Autodesk Fusion 360 part; units mm, degrees
(part 2 of 12)
  line L834 (3.1315, 118.2846) -> (7.4616, 115.7846)
  line L835 (7.4616, 115.7846) -> (11.7918, 118.2846)
  line L836 (11.7918, 118.2846) -> (11.7918, 123.2846)
  line L837 (11.7918, 123.2846) -> (7.4616, 125.7846)
  line L838 (18.1219, 125.7846) -> (13.7918, 123.2846)
  line L839 (13.7918, 123.2846) -> (13.7918, 118.2846)
  line L840 (13.7918, 118.2846) -> (18.1219, 115.7846)
  line L841 (18.1219, 115.7846) -> (22.452, 118.2846)
  line L842 (22.452, 118.2846) -> (22.452, 123.2846)
  line L843 (22.452, 123.2846) -> (18.1219, 125.7846)
  line L844 (28.7821, 125.7846) -> (24.452, 123.2846)
  line L845 (24.452, 123.2846) -> (24.452, 118.2846)
  line L846 (24.452, 118.2846) -> (28.7821, 115.7846)
  line L847 (28.7821, 115.7846) -> (33.1123, 118.2846)
  line L848 (33.1123, 118.2846) -> (33.1123, 123.2846)
  line L849 (33.1123, 123.2846) -> (28.7821, 125.7846)
  line L850 (39.4424, 125.7846) -> (35.1123, 123.2846)
  line L851 (35.1123, 123.2846) -> (35.1123, 118.2846)
  line L852 (35.1123, 118.2846) -> (39.4424, 115.7846)
  line L853 (39.4424, 115.7846) -> (43.7725, 118.2846)
  line L854 (43.7725, 118.2846) -> (43.7725, 123.2846)
  line L855 (43.7725, 123.2846) -> (39.4424, 125.7846)
  line L856 (50.1027, 125.7846) -> (45.7725, 123.2846)
  line L857 (45.7725, 123.2846) -> (45.7725, 118.2846)
  line L858 (45.7725, 118.2846) -> (50.1027, 115.7846)
  line L859 (50.1027, 115.7846) -> (54.4328, 118.2846)
  line L860 (54.4328, 118.2846) -> (54.4328, 123.2846)
  line L861 (54.4328, 123.2846) -> (50.1027, 125.7846)
  line L862 (-51.1698, 135.0167) -> (-55.4999, 132.5167)
  line L863 (-55.4999, 132.5167) -> (-55.4999, 127.5167)
  line L864 (-55.4999, 127.5167) -> (-51.1698, 125.0167)
  line L865 (-51.1698, 125.0167) -> (-46.8396, 127.5167)
  line L866 (-46.8396, 127.5167) -> (-46.8396, 132.5167)
  line L867 (-46.8396, 132.5167) -> (-51.1698, 135.0167)
  line L868 (-40.5095, 135.0167) -> (-44.8396, 132.5167)
  line L869 (-44.8396, 132.5167) -> (-44.8396, 127.5167)
  line L870 (-44.8396, 127.5167) -> (-40.5095, 125.0167)
  line L871 (-40.5095, 125.0167) -> (-36.1794, 127.5167)
  line L872 (-36.1794, 127.5167) -> (-36.1794, 132.5167)
  line L873 (-36.1794, 132.5167) -> (-40.5095, 135.0167)
  line L874 (-29.8493, 135.0167) -> (-34.1794, 132.5167)
  line L875 (-34.1794, 132.5167) -> (-34.1794, 127.5167)
  line L876 (-34.1794, 127.5167) -> (-29.8493, 125.0167)
  line L877 (-29.8493, 125.0167) -> (-25.5191, 127.5167)
  line L878 (-25.5191, 127.5167) -> (-25.5191, 132.5167)
  line L879 (-25.5191, 132.5167) -> (-29.8493, 135.0167)
  line L880 (-19.189, 135.0167) -> (-23.5191, 132.5167)
  line L881 (-23.5191, 132.5167) -> (-23.5191, 127.5167)
  line L882 (-23.5191, 127.5167) -> (-19.189, 125.0167)
  line L883 (-19.189, 125.0167) -> (-14.8589, 127.5167)
  line L884 (-14.8589, 127.5167) -> (-14.8589, 132.5167)
  line L885 (-14.8589, 132.5167) -> (-19.189, 135.0167)
  line L886 (-8.5287, 135.0167) -> (-12.8589, 132.5167)
  line L887 (-12.8589, 132.5167) -> (-12.8589, 127.5167)
  line L888 (-12.8589, 127.5167) -> (-8.5287, 125.0167)
  line L889 (-8.5287, 125.0167) -> (-4.1986, 127.5167)
  line L890 (-4.1986, 127.5167) -> (-4.1986, 132.5167)
  line L891 (-4.1986, 132.5167) -> (-8.5287, 135.0167)
  line L892 (2.1315, 135.0167) -> (-2.1986, 132.5167)
  line L893 (-2.1986, 132.5167) -> (-2.1986, 127.5167)
  line L894 (-2.1986, 127.5167) -> (2.1315, 125.0167)
  line L895 (2.1315, 125.0167) -> (6.4616, 127.5167)
  line L896 (6.4616, 127.5167) -> (6.4616, 132.5167)
  line L897 (6.4616, 132.5167) -> (2.1315, 135.0167)
  line L898 (12.7918, 135.0167) -> (8.4616, 132.5167)
  line L899 (8.4616, 132.5167) -> (8.4616, 127.5167)
  line L900 (8.4616, 127.5167) -> (12.7918, 125.0167)
  line L901 (12.7918, 125.0167) -> (17.1219, 127.5167)
  line L902 (17.1219, 127.5167) -> (17.1219, 132.5167)
  line L903 (17.1219, 132.5167) -> (12.7918, 135.0167)
  line L904 (23.452, 135.0167) -> (19.1219, 132.5167)
  line L905 (19.1219, 132.5167) -> (19.1219, 127.5167)
  line L906 (19.1219, 127.5167) -> (23.452, 125.0167)
  line L907 (23.452, 125.0167) -> (27.7821, 127.5167)
  line L908 (27.7821, 127.5167) -> (27.7821, 132.5167)
  line L909 (27.7821, 132.5167) -> (23.452, 135.0167)
  line L910 (34.1123, 135.0167) -> (29.7821, 132.5167)
  line L911 (29.7821, 132.5167) -> (29.7821, 127.5167)
  line L912 (29.7821, 127.5167) -> (34.1123, 125.0167)
  line L913 (34.1123, 125.0167) -> (38.4424, 127.5167)
  line L914 (38.4424, 127.5167) -> (38.4424, 132.5167)
  line L915 (38.4424, 132.5167) -> (34.1123, 135.0167)
  line L916 (44.7725, 135.0167) -> (40.4424, 132.5167)
  line L917 (40.4424, 132.5167) -> (40.4424, 127.5167)
  line L918 (40.4424, 127.5167) -> (44.7725, 125.0167)
  line L919 (44.7725, 125.0167) -> (49.1027, 127.5167)
  line L920 (49.1027, 127.5167) -> (49.1027, 132.5167)
  line L921 (49.1027, 132.5167) -> (44.7725, 135.0167)
  line L922 (55.4328, 135.0167) -> (51.1027, 132.5167)
  line L923 (51.1027, 132.5167) -> (51.1027, 127.5167)
  line L924 (51.1027, 127.5167) -> (55.4328, 125.0167)
  line L925 (55.4328, 125.0167) -> (59.7629, 127.5167)
  line L926 (59.7629, 127.5167) -> (59.7629, 132.5167)
  line L927 (59.7629, 132.5167) -> (55.4328, 135.0167)
  line L928 (-56.4999, 144.2487) -> (-60.83, 141.7487)
  line L929 (-60.83, 141.7487) -> (-60.83, 136.7487)
  line L930 (-60.83, 136.7487) -> (-56.4999, 134.2487)
  line L931 (-56.4999, 134.2487) -> (-52.1698, 136.7487)
  line L932 (-52.1698, 136.7487) -> (-52.1698, 141.7487)
  line L933 (-52.1698, 141.7487) -> (-56.4999, 144.2487)
  line L934 (-45.8396, 144.2487) -> (-50.1698, 141.7487)
  line L935 (-50.1698, 141.7487) -> (-50.1698, 136.7487)
  line L936 (-50.1698, 136.7487) -> (-45.8396, 134.2487)
  line L937 (-45.8396, 134.2487) -> (-41.5095, 136.7487)
  line L938 (-41.5095, 136.7487) -> (-41.5095, 141.7487)
  line L939 (-41.5095, 141.7487) -> (-45.8396, 144.2487)
  line L940 (-35.1794, 144.2487) -> (-39.5095, 141.7487)
  line L941 (-39.5095, 141.7487) -> (-39.5095, 136.7487)
  line L942 (-39.5095, 136.7487) -> (-35.1794, 134.2487)
  line L943 (-35.1794, 134.2487) -> (-30.8493, 136.7487)
  line L944 (-30.8493, 136.7487) -> (-30.8493, 141.7487)
  line L945 (-30.8493, 141.7487) -> (-35.1794, 144.2487)
  line L946 (-24.5191, 144.2487) -> (-28.8493, 141.7487)
  line L947 (-28.8493, 141.7487) -> (-28.8493, 136.7487)
  line L948 (-28.8493, 136.7487) -> (-24.5191, 134.2487)
  line L949 (-24.5191, 134.2487) -> (-20.189, 136.7487)
  line L950 (-20.189, 136.7487) -> (-20.189, 141.7487)
  line L951 (-20.189, 141.7487) -> (-24.5191, 144.2487)
  line L952 (-13.8589, 144.2487) -> (-18.189, 141.7487)
  line L953 (-18.189, 141.7487) -> (-18.189, 136.7487)
  line L954 (-18.189, 136.7487) -> (-13.8589, 134.2487)
  line L955 (-13.8589, 134.2487) -> (-9.5287, 136.7487)
  line L956 (-9.5287, 136.7487) -> (-9.5287, 141.7487)
  line L957 (-9.5287, 141.7487) -> (-13.8589, 144.2487)
  line L958 (-3.1986, 144.2487) -> (-7.5287, 141.7487)
  line L959 (-7.5287, 141.7487) -> (-7.5287, 136.7487)
  line L960 (-7.5287, 136.7487) -> (-3.1986, 134.2487)
  line L961 (-3.1986, 134.2487) -> (1.1315, 136.7487)
  line L962 (1.1315, 136.7487) -> (1.1315, 141.7487)
  line L963 (1.1315, 141.7487) -> (-3.1986, 144.2487)
  line L964 (7.4616, 144.2487) -> (3.1315, 141.7487)
  line L965 (3.1315, 141.7487) -> (3.1315, 136.7487)
  line L966 (3.1315, 136.7487) -> (7.4616, 134.2487)
  line L967 (7.4616, 134.2487) -> (11.7918, 136.7487)
  line L968 (11.7918, 136.7487) -> (11.7918, 141.7487)
  line L969 (11.7918, 141.7487) -> (7.4616, 144.2487)
  line L970 (18.1219, 144.2487) -> (13.7918, 141.7487)
  line L971 (13.7918, 141.7487) -> (13.7918, 136.7487)
  line L972 (13.7918, 136.7487) -> (18.1219, 134.2487)
  line L973 (18.1219, 134.2487) -> (22.452, 136.7487)
  line L974 (22.452, 136.7487) -> (22.452, 141.7487)
  line L975 (22.452, 141.7487) -> (18.1219, 144.2487)
  line L976 (28.7821, 144.2487) -> (24.452, 141.7487)
  line L977 (24.452, 141.7487) -> (24.452, 136.7487)
  line L978 (24.452, 136.7487) -> (28.7821, 134.2487)
  line L979 (28.7821, 134.2487) -> (33.1123, 136.7487)
  line L980 (33.1123, 136.7487) -> (33.1123, 141.7487)
  line L981 (33.1123, 141.7487) -> (28.7821, 144.2487)
  line L982 (39.4424, 144.2487) -> (35.1123, 141.7487)
  line L983 (35.1123, 141.7487) -> (35.1123, 136.7487)
  line L984 (35.1123, 136.7487) -> (39.4424, 134.2487)
  line L985 (39.4424, 134.2487) -> (43.7725, 136.7487)
  line L986 (43.7725, 136.7487) -> (43.7725, 141.7487)
  line L987 (43.7725, 141.7487) -> (39.4424, 144.2487)
  line L988 (50.1027, 144.2487) -> (45.7725, 141.7487)
  line L989 (45.7725, 141.7487) -> (45.7725, 136.7487)
  line L990 (45.7725, 136.7487) -> (50.1027, 134.2487)
  line L991 (50.1027, 134.2487) -> (54.4328, 136.7487)
  line L992 (54.4328, 136.7487) -> (54.4328, 141.7487)
  line L993 (54.4328, 141.7487) -> (50.1027, 144.2487)
  line L994 (-51.1698, 153.4808) -> (-55.4999, 150.9808)
  line L995 (-55.4999, 150.9808) -> (-55.4999, 145.9808)
  line L996 (-55.4999, 145.9808) -> (-51.1698, 143.4808)
  line L997 (-51.1698, 143.4808) -> (-46.8396, 145.9808)
  line L998 (-46.8396, 145.9808) -> (-46.8396, 150.9808)
  line L999 (-46.8396, 150.9808) -> (-51.1698, 153.4808)
  line L1000 (-40.5095, 153.4808) -> (-44.8396, 150.9808)
  line L1001 (-44.8396, 150.9808) -> (-44.8396, 145.9808)
  line L1002 (-44.8396, 145.9808) -> (-40.5095, 143.4808)
  line L1003 (-40.5095, 143.4808) -> (-36.1794, 145.9808)
  line L1004 (-36.1794, 145.9808) -> (-36.1794, 150.9808)
  line L1005 (-36.1794, 150.9808) -> (-40.5095, 153.4808)
  line L1006 (-29.8493, 153.4808) -> (-34.1794, 150.9808)
  line L1007 (-34.1794, 150.9808) -> (-34.1794, 145.9808)
  line L1008 (-34.1794, 145.9808) -> (-29.8493, 143.4808)
  line L1009 (-29.8493, 143.4808) -> (-25.5191, 145.9808)
  line L1010 (-25.5191, 145.9808) -> (-25.5191, 150.9808)
  line L1011 (-25.5191, 150.9808) -> (-29.8493, 153.4808)
  line L1012 (-19.189, 153.4808) -> (-23.5191, 150.9808)
  line L1013 (-23.5191, 150.9808) -> (-23.5191, 145.9808)
  line L1014 (-23.5191, 145.9808) -> (-19.189, 143.4808)
  line L1015 (-19.189, 143.4808) -> (-14.8589, 145.9808)
  line L1016 (-14.8589, 145.9808) -> (-14.8589, 150.9808)
  line L1017 (-14.8589, 150.9808) -> (-19.189, 153.4808)
  line L1018 (-8.5287, 153.4808) -> (-12.8589, 150.9808)
  line L1019 (-12.8589, 150.9808) -> (-12.8589, 145.9808)
  line L1020 (-12.8589, 145.9808) -> (-8.5287, 143.4808)
  line L1021 (-8.5287, 143.4808) -> (-4.1986, 145.9808)
  line L1022 (-4.1986, 145.9808) -> (-4.1986, 150.9808)
  line L1023 (-4.1986, 150.9808) -> (-8.5287, 153.4808)
  line L1024 (2.1315, 153.4808) -> (-2.1986, 150.9808)
  line L1025 (-2.1986, 150.9808) -> (-2.1986, 145.9808)
  line L1026 (-2.1986, 145.9808) -> (2.1315, 143.4808)
  line L1027 (2.1315, 143.4808) -> (6.4616, 145.9808)
  line L1028 (6.4616, 145.9808) -> (6.4616, 150.9808)
  line L1029 (6.4616, 150.9808) -> (2.1315, 153.4808)
  line L1030 (12.7918, 153.4808) -> (8.4616, 150.9808)
  line L1031 (8.4616, 150.9808) -> (8.4616, 145.9808)
  line L1032 (8.4616, 145.9808) -> (12.7918, 143.4808)
  line L1033 (12.7918, 143.4808) -> (17.1219, 145.9808)
  line L1034 (17.1219, 145.9808) -> (17.1219, 150.9808)
  line L1035 (17.1219, 150.9808) -> (12.7918, 153.4808)
  line L1036 (23.452, 153.4808) -> (19.1219, 150.9808)
  line L1037 (19.1219, 150.9808) -> (19.1219, 145.9808)
  line L1038 (19.1219, 145.9808) -> (23.452, 143.4808)
  line L1039 (23.452, 143.4808) -> (27.7821, 145.9808)
  line L1040 (27.7821, 145.9808) -> (27.7821, 150.9808)
  line L1041 (27.7821, 150.9808) -> (23.452, 153.4808)
  line L1042 (34.1123, 153.4808) -> (29.7821, 150.9808)
  line L1043 (29.7821, 150.9808) -> (29.7821, 145.9808)
  line L1044 (29.7821, 145.9808) -> (34.1123, 143.4808)
  line L1045 (34.1123, 143.4808) -> (38.4424, 145.9808)
  line L1046 (38.4424, 145.9808) -> (38.4424, 150.9808)
  line L1047 (38.4424, 150.9808) -> (34.1123, 153.4808)
  line L1048 (44.7725, 153.4808) -> (40.4424, 150.9808)
  line L1049 (40.4424, 150.9808) -> (40.4424, 145.9808)
  line L1050 (40.4424, 145.9808) -> (44.7725, 143.4808)
  line L1051 (44.7725, 143.4808) -> (49.1027, 145.9808)
  line L1052 (49.1027, 145.9808) -> (49.1027, 150.9808)
  line L1053 (49.1027, 150.9808) -> (44.7725, 153.4808)
  line L1054 (55.4328, 153.4808) -> (51.1027, 150.9808)
  line L1055 (51.1027, 150.9808) -> (51.1027, 145.9808)
  line L1056 (51.1027, 145.9808) -> (55.4328, 143.4808)
  line L1057 (55.4328, 143.4808) -> (59.7629, 145.9808)
  line L1058 (59.7629, 145.9808) -> (59.7629, 150.9808)
  line L1059 (59.7629, 150.9808) -> (55.4328, 153.4808)
  line L1060 (-56.4999, 162.7128) -> (-60.83, 160.2128)
  line L1061 (-60.83, 160.2128) -> (-60.83, 155.2128)
  line L1062 (-60.83, 155.2128) -> (-56.4999, 152.7128)
  line L1063 (-56.4999, 152.7128) -> (-52.1698, 155.2128)
  line L1064 (-52.1698, 155.2128) -> (-52.1698, 160.2128)
  line L1065 (-52.1698, 160.2128) -> (-56.4999, 162.7128)
  line L1066 (-45.8396, 162.7128) -> (-50.1698, 160.2128)
  line L1067 (-50.1698, 160.2128) -> (-50.1698, 155.2128)
  line L1068 (-50.1698, 155.2128) -> (-45.8396, 152.7128)
  line L1069 (-45.8396, 152.7128) -> (-41.5095, 155.2128)
  line L1070 (-41.5095, 155.2128) -> (-41.5095, 160.2128)
  line L1071 (-41.5095, 160.2128) -> (-45.8396, 162.7128)
  line L1072 (-35.1794, 162.7128) -> (-39.5095, 160.2128)
  line L1073 (-39.5095, 160.2128) -> (-39.5095, 155.2128)
  line L1074 (-39.5095, 155.2128) -> (-35.1794, 152.7128)
  line L1075 (-35.1794, 152.7128) -> (-30.8493, 155.2128)
  line L1076 (-30.8493, 155.2128) -> (-30.8493, 160.2128)
  line L1077 (-30.8493, 160.2128) -> (-35.1794, 162.7128)
  line L1078 (-24.5191, 162.7128) -> (-28.8493, 160.2128)
  line L1079 (-28.8493, 160.2128) -> (-28.8493, 155.2128)
  line L1080 (-28.8493, 155.2128) -> (-24.5191, 152.7128)
  line L1081 (-24.5191, 152.7128) -> (-20.189, 155.2128)
  line L1082 (-20.189, 155.2128) -> (-20.189, 160.2128)
  line L1083 (-20.189, 160.2128) -> (-24.5191, 162.7128)
  line L1084 (-13.8589, 162.7128) -> (-18.189, 160.2128)
  line L1085 (-18.189, 160.2128) -> (-18.189, 155.2128)
  line L1086 (-18.189, 155.2128) -> (-13.8589, 152.7128)
  line L1087 (-13.8589, 152.7128) -> (-9.5287, 155.2128)
  line L1088 (-9.5287, 155.2128) -> (-9.5287, 160.2128)
  line L1089 (-9.5287, 160.2128) -> (-13.8589, 162.7128)
  line L1090 (-3.1986, 162.7128) -> (-7.5287, 160.2128)
  line L1091 (-7.5287, 160.2128) -> (-7.5287, 155.2128)
  line L1092 (-7.5287, 155.2128) -> (-3.1986, 152.7128)
  line L1093 (-3.1986, 152.7128) -> (1.1315, 155.2128)
  line L1094 (1.1315, 155.2128) -> (1.1315, 160.2128)
  line L1095 (1.1315, 160.2128) -> (-3.1986, 162.7128)
  line L1096 (7.4616, 162.7128) -> (3.1315, 160.2128)
  line L1097 (3.1315, 160.2128) -> (3.1315, 155.2128)
  line L1098 (3.1315, 155.2128) -> (7.4616, 152.7128)
  line L1099 (7.4616, 152.7128) -> (11.7918, 155.2128)
  line L1100 (11.7918, 155.2128) -> (11.7918, 160.2128)
  line L1101 (11.7918, 160.2128) -> (7.4616, 162.7128)
  line L1102 (18.1219, 162.7128) -> (13.7918, 160.2128)
  line L1103 (13.7918, 160.2128) -> (13.7918, 155.2128)
  line L1104 (13.7918, 155.2128) -> (18.1219, 152.7128)
  line L1105 (18.1219, 152.7128) -> (22.452, 155.2128)
  line L1106 (22.452, 155.2128) -> (22.452, 160.2128)
  line L1107 (22.452, 160.2128) -> (18.1219, 162.7128)
  line L1108 (28.7821, 162.7128) -> (24.452, 160.2128)
  line L1109 (24.452, 160.2128) -> (24.452, 155.2128)
  line L1110 (24.452, 155.2128) -> (28.7821, 152.7128)
  line L1111 (28.7821, 152.7128) -> (33.1123, 155.2128)
  line L1112 (33.1123, 155.2128) -> (33.1123, 160.2128)
  line L1113 (33.1123, 160.2128) -> (28.7821, 162.7128)
  line L1114 (39.4424, 162.7128) -> (35.1123, 160.2128)
  line L1115 (35.1123, 160.2128) -> (35.1123, 155.2128)
  line L1116 (35.1123, 155.2128) -> (39.4424, 152.7128)
  line L1117 (39.4424, 152.7128) -> (43.7725, 155.2128)
  line L1118 (43.7725, 155.2128) -> (43.7725, 160.2128)
  line L1119 (43.7725, 160.2128) -> (39.4424, 162.7128)
  line L1120 (50.1027, 162.7128) -> (45.7725, 160.2128)
  line L1121 (45.7725, 160.2128) -> (45.7725, 155.2128)
  line L1122 (45.7725, 155.2128) -> (50.1027, 152.7128)
  line L1123 (50.1027, 152.7128) -> (54.4328, 155.2128)
  line L1124 (54.4328, 155.2128) -> (54.4328, 160.2128)
  line L1125 (54.4328, 160.2128) -> (50.1027, 162.7128)
  line L1126 (-51.1698, 171.9449) -> (-55.4999, 169.4449)
  line L1127 (-55.4999, 169.4449) -> (-55.4999, 164.4449)
  line L1128 (-55.4999, 164.4449) -> (-51.1698, 161.9449)
  line L1129 (-51.1698, 161.9449) -> (-46.8396, 164.4449)
  line L1130 (-46.8396, 164.4449) -> (-46.8396, 169.4449)
  line L1131 (-46.8396, 169.4449) -> (-51.1698, 171.9449)
  line L1132 (-40.5095, 171.9449) -> (-44.8396, 169.4449)
  line L1133 (-44.8396, 169.4449) -> (-44.8396, 164.4449)
  line L1134 (-44.8396, 164.4449) -> (-40.5095, 161.9449)
  line L1135 (-40.5095, 161.9449) -> (-36.1794, 164.4449)
  line L1136 (-36.1794, 164.4449) -> (-36.1794, 169.4449)
  line L1137 (-36.1794, 169.4449) -> (-40.5095, 171.9449)
  line L1138 (-29.8493, 171.9449) -> (-34.1794, 169.4449)
  line L1139 (-34.1794, 169.4449) -> (-34.1794, 164.4449)
  line L1140 (-34.1794, 164.4449) -> (-29.8493, 161.9449)
  line L1141 (-29.8493, 161.9449) -> (-25.5191, 164.4449)
  line L1142 (-25.5191, 164.4449) -> (-25.5191, 169.4449)
  line L1143 (-25.5191, 169.4449) -> (-29.8493, 171.9449)
  line L1144 (-19.189, 171.9449) -> (-23.5191, 169.4449)
  line L1145 (-23.5191, 169.4449) -> (-23.5191, 164.4449)
  line L1146 (-23.5191, 164.4449) -> (-19.189, 161.9449)
  line L1147 (-19.189, 161.9449) -> (-14.8589, 164.4449)
  line L1148 (-14.8589, 164.4449) -> (-14.8589, 169.4449)
  line L1149 (-14.8589, 169.4449) -> (-19.189, 171.9449)
  line L1150 (-8.5287, 171.9449) -> (-12.8589, 169.4449)
  line L1151 (-12.8589, 169.4449) -> (-12.8589, 164.4449)
  line L1152 (-12.8589, 164.4449) -> (-8.5287, 161.9449)
  line L1153 (-8.5287, 161.9449) -> (-4.1986, 164.4449)
  line L1154 (-4.1986, 164.4449) -> (-4.1986, 169.4449)
  line L1155 (-4.1986, 169.4449) -> (-8.5287, 171.9449)
  line L1156 (2.1315, 171.9449) -> (-2.1986, 169.4449)
  line L1157 (-2.1986, 169.4449) -> (-2.1986, 164.4449)
  line L1158 (-2.1986, 164.4449) -> (2.1315, 161.9449)
  line L1159 (2.1315, 161.9449) -> (6.4616, 164.4449)
  line L1160 (6.4616, 164.4449) -> (6.4616, 169.4449)
  line L1161 (6.4616, 169.4449) -> (2.1315, 171.9449)
  line L1162 (12.7918, 171.9449) -> (8.4616, 169.4449)
  line L1163 (8.4616, 169.4449) -> (8.4616, 164.4449)
  line L1164 (8.4616, 164.4449) -> (12.7918, 161.9449)
  line L1165 (12.7918, 161.9449) -> (17.1219, 164.4449)
  line L1166 (17.1219, 164.4449) -> (17.1219, 169.4449)
  line L1167 (17.1219, 169.4449) -> (12.7918, 171.9449)
  line L1168 (23.452, 171.9449) -> (19.1219, 169.4449)
  line L1169 (19.1219, 169.4449) -> (19.1219, 164.4449)
  line L1170 (19.1219, 164.4449) -> (23.452, 161.9449)
  line L1171 (23.452, 161.9449) -> (27.7821, 164.4449)
  line L1172 (27.7821, 164.4449) -> (27.7821, 169.4449)
  line L1173 (27.7821, 169.4449) -> (23.452, 171.9449)
  line L1174 (34.1123, 171.9449) -> (29.7821, 169.4449)
  line L1175 (29.7821, 169.4449) -> (29.7821, 164.4449)
  line L1176 (29.7821, 164.4449) -> (34.1123, 161.9449)
  line L1177 (34.1123, 161.9449) -> (38.4424, 164.4449)
  line L1178 (38.4424, 164.4449) -> (38.4424, 169.4449)
  line L1179 (38.4424, 169.4449) -> (34.1123, 171.9449)
  line L1180 (44.7725, 171.9449) -> (40.4424, 169.4449)
  line L1181 (40.4424, 169.4449) -> (40.4424, 164.4449)
  line L1182 (40.4424, 164.4449) -> (44.7725, 161.9449)
  line L1183 (44.7725, 161.9449) -> (49.1027, 164.4449)
  line L1184 (49.1027, 164.4449) -> (49.1027, 169.4449)
  line L1185 (49.1027, 169.4449) -> (44.7725, 171.9449)
  line L1186 (55.4328, 171.9449) -> (51.1027, 169.4449)
  line L1187 (51.1027, 169.4449) -> (51.1027, 164.4449)
  line L1188 (51.1027, 164.4449) -> (55.4328, 161.9449)
  line L1189 (55.4328, 161.9449) -> (59.7629, 164.4449)
  line L1190 (59.7629, 164.4449) -> (59.7629, 169.4449)
  line L1191 (59.7629, 169.4449) -> (55.4328, 171.9449)
  line L1192 (-56.4999, 181.1769) -> (-60.83, 178.6769)
  line L1193 (-60.83, 178.6769) -> (-60.83, 173.6769)
  line L1194 (-60.83, 173.6769) -> (-56.4999, 171.1769)
  line L1195 (-56.4999, 171.1769) -> (-52.1698, 173.6769)
  line L1196 (-52.1698, 173.6769) -> (-52.1698, 178.6769)
  line L1197 (-52.1698, 178.6769) -> (-56.4999, 181.1769)
  line L1198 (-45.8396, 181.1769) -> (-50.1698, 178.6769)
  line L1199 (-50.1698, 178.6769) -> (-50.1698, 173.6769)
  line L1200 (-50.1698, 173.6769) -> (-45.8396, 171.1769)
  line L1201 (-45.8396, 171.1769) -> (-41.5095, 173.6769)
  line L1202 (-41.5095, 173.6769) -> (-41.5095, 178.6769)
  line L1203 (-41.5095, 178.6769) -> (-45.8396, 181.1769)
  line L1204 (-35.1794, 181.1769) -> (-39.5095, 178.6769)
  line L1205 (-39.5095, 178.6769) -> (-39.5095, 173.6769)
  line L1206 (-39.5095, 173.6769) -> (-35.1794, 171.1769)
  line L1207 (-35.1794, 171.1769) -> (-30.8493, 173.6769)
  line L1208 (-30.8493, 173.6769) -> (-30.8493, 178.6769)
  line L1209 (-30.8493, 178.6769) -> (-35.1794, 181.1769)
  line L1210 (-24.5191, 181.1769) -> (-28.8493, 178.6769)
  line L1211 (-28.8493, 178.6769) -> (-28.8493, 173.6769)
  line L1212 (-28.8493, 173.6769) -> (-24.5191, 171.1769)
  line L1213 (-24.5191, 171.1769) -> (-20.189, 173.6769)
  line L1214 (-20.189, 173.6769) -> (-20.189, 178.6769)
  line L1215 (-20.189, 178.6769) -> (-24.5191, 181.1769)
  line L1216 (-13.8589, 181.1769) -> (-18.189, 178.6769)
  line L1217 (-18.189, 178.6769) -> (-18.189, 173.6769)
  line L1218 (-18.189, 173.6769) -> (-13.8589, 171.1769)
  line L1219 (-13.8589, 171.1769) -> (-9.5287, 173.6769)
  line L1220 (-9.5287, 173.6769) -> (-9.5287, 178.6769)
  line L1221 (-9.5287, 178.6769) -> (-13.8589, 181.1769)
  line L1222 (-3.1986, 181.1769) -> (-7.5287, 178.6769)
  line L1223 (-7.5287, 178.6769) -> (-7.5287, 173.6769)
  line L1224 (-7.5287, 173.6769) -> (-3.1986, 171.1769)
  line L1225 (-3.1986, 171.1769) -> (1.1315, 173.6769)
  line L1226 (1.1315, 173.6769) -> (1.1315, 178.6769)
  line L1227 (1.1315, 178.6769) -> (-3.1986, 181.1769)
  line L1228 (7.4616, 181.1769) -> (3.1315, 178.6769)
  line L1229 (3.1315, 178.6769) -> (3.1315, 173.6769)
  line L1230 (3.1315, 173.6769) -> (7.4616, 171.1769)
  line L1231 (7.4616, 171.1769) -> (11.7918, 173.6769)
  line L1232 (11.7918, 173.6769) -> (11.7918, 178.6769)
  line L1233 (11.7918, 178.6769) -> (7.4616, 181.1769)
  line L1234 (18.1219, 181.1769) -> (13.7918, 178.6769)
  line L1235 (13.7918, 178.6769) -> (13.7918, 173.6769)
  line L1236 (13.7918, 173.6769) -> (18.1219, 171.1769)
  line L1237 (18.1219, 171.1769) -> (22.452, 173.6769)
  line L1238 (22.452, 173.6769) -> (22.452, 178.6769)
  line L1239 (22.452, 178.6769) -> (18.1219, 181.1769)
  line L1240 (28.7821, 181.1769) -> (24.452, 178.6769)
  line L1241 (24.452, 178.6769) -> (24.452, 173.6769)
  line L1242 (24.452, 173.6769) -> (28.7821, 171.1769)
  line L1243 (28.7821, 171.1769) -> (33.1123, 173.6769)
  line L1244 (33.1123, 173.6769) -> (33.1123, 178.6769)
  line L1245 (33.1123, 178.6769) -> (28.7821, 181.1769)
  line L1246 (39.4424, 181.1769) -> (35.1123, 178.6769)
  line L1247 (35.1123, 178.6769) -> (35.1123, 173.6769)
  line L1248 (35.1123, 173.6769) -> (39.4424, 171.1769)
  line L1249 (39.4424, 171.1769) -> (43.7725, 173.6769)
  line L1250 (43.7725, 173.6769) -> (43.7725, 178.6769)
  line L1251 (43.7725, 178.6769) -> (39.4424, 181.1769)
  line L1252 (50.1027, 181.1769) -> (45.7725, 178.6769)
  line L1253 (45.7725, 178.6769) -> (45.7725, 173.6769)
  line L1254 (45.7725, 173.6769) -> (50.1027, 171.1769)
  line L1255 (50.1027, 171.1769) -> (54.4328, 173.6769)
  line L1256 (54.4328, 173.6769) -> (54.4328, 178.6769)
  line L1257 (54.4328, 178.6769) -> (50.1027, 181.1769)
  line L1258 (-51.1698, 190.409) -> (-55.4999, 187.909)
  line L1259 (-55.4999, 187.909) -> (-55.4999, 182.909)
  line L1260 (-55.4999, 182.909) -> (-51.1698, 180.409)
  line L1261 (-51.1698, 180.409) -> (-46.8396, 182.909)
  line L1262 (-46.8396, 182.909) -> (-46.8396, 187.909)
  line L1263 (-46.8396, 187.909) -> (-51.1698, 190.409)
  line L1264 (-40.5095, 190.409) -> (-44.8396, 187.909)
  line L1265 (-44.8396, 187.909) -> (-44.8396, 182.909)
  line L1266 (-44.8396, 182.909) -> (-40.5095, 180.409)
  line L1267 (-40.5095, 180.409) -> (-36.1794, 182.909)
  line L1268 (-36.1794, 182.909) -> (-36.1794, 187.909)
  line L1269 (-36.1794, 187.909) -> (-40.5095, 190.409)
  line L1270 (-29.8493, 190.409) -> (-34.1794, 187.909)
  line L1271 (-34.1794, 187.909) -> (-34.1794, 182.909)
  line L1272 (-34.1794, 182.909) -> (-29.8493, 180.409)
  line L1273 (-29.8493, 180.409) -> (-25.5191, 182.909)
  line L1274 (-25.5191, 182.909) -> (-25.5191, 187.909)
  line L1275 (-25.5191, 187.909) -> (-29.8493, 190.409)
  line L1276 (-19.189, 190.409) -> (-23.5191, 187.909)
  line L1277 (-23.5191, 187.909) -> (-23.5191, 182.909)
  line L1278 (-23.5191, 182.909) -> (-19.189, 180.409)
  line L1279 (-19.189, 180.409) -> (-14.8589, 182.909)
  line L1280 (-14.8589, 182.909) -> (-14.8589, 187.909)
  line L1281 (-14.8589, 187.909) -> (-19.189, 190.409)
  line L1282 (-8.5287, 190.409) -> (-12.8589, 187.909)
  line L1283 (-12.8589, 187.909) -> (-12.8589, 182.909)
  line L1284 (-12.8589, 182.909) -> (-8.5287, 180.409)
  line L1285 (-8.5287, 180.409) -> (-4.1986, 182.909)
  line L1286 (-4.1986, 182.909) -> (-4.1986, 187.909)
  line L1287 (-4.1986, 187.909) -> (-8.5287, 190.409)
  line L1288 (2.1315, 190.409) -> (-2.1986, 187.909)
  line L1289 (-2.1986, 187.909) -> (-2.1986, 182.909)
  line L1290 (-2.1986, 182.909) -> (2.1315, 180.409)
  line L1291 (2.1315, 180.409) -> (6.4616, 182.909)
  line L1292 (6.4616, 182.909) -> (6.4616, 187.909)
  line L1293 (6.4616, 187.909) -> (2.1315, 190.409)
  line L1294 (12.7918, 190.409) -> (8.4616, 187.909)
  line L1295 (8.4616, 187.909) -> (8.4616, 182.909)
  line L1296 (8.4616, 182.909) -> (12.7918, 180.409)
  line L1297 (12.7918, 180.409) -> (17.1219, 182.909)
  line L1298 (17.1219, 182.909) -> (17.1219, 187.909)
  line L1299 (17.1219, 187.909) -> (12.7918, 190.409)
  line L1300 (23.452, 190.409) -> (19.1219, 187.909)
  line L1301 (19.1219, 187.909) -> (19.1219, 182.909)
  line L1302 (19.1219, 182.909) -> (23.452, 180.409)
  line L1303 (23.452, 180.409) -> (27.7821, 182.909)
  line L1304 (27.7821, 182.909) -> (27.7821, 187.909)
  line L1305 (27.7821, 187.909) -> (23.452, 190.409)
  line L1306 (34.1123, 190.409) -> (29.7821, 187.909)
  line L1307 (29.7821, 187.909) -> (29.7821, 182.909)
  line L1308 (29.7821, 182.909) -> (34.1123, 180.409)
  line L1309 (34.1123, 180.409) -> (38.4424, 182.909)
  line L1310 (38.4424, 182.909) -> (38.4424, 187.909)
  line L1311 (38.4424, 187.909) -> (34.1123, 190.409)
  line L1312 (44.7725, 190.409) -> (40.4424, 187.909)
  line L1313 (40.4424, 187.909) -> (40.4424, 182.909)
  line L1314 (40.4424, 182.909) -> (44.7725, 180.409)
  line L1315 (44.7725, 180.409) -> (49.1027, 182.909)
  line L1316 (49.1027, 182.909) -> (49.1027, 187.909)
  line L1317 (49.1027, 187.909) -> (44.7725, 190.409)
  line L1318 (55.4328, 190.409) -> (51.1027, 187.909)
  line L1319 (51.1027, 187.909) -> (51.1027, 182.909)
  line L1320 (51.1027, 182.909) -> (55.4328, 180.409)
  line L1321 (55.4328, 180.409) -> (59.7629, 182.909)
  line L1322 (59.7629, 182.909) -> (59.7629, 187.909)
  line L1323 (59.7629, 187.909) -> (55.4328, 190.409)
  line L1324 (-56.4999, 199.641) -> (-60.83, 197.141)
  line L1325 (-60.83, 197.141) -> (-60.83, 192.141)
  line L1326 (-60.83, 192.141) -> (-56.4999, 189.641)
  line L1327 (-56.4999, 189.641) -> (-52.1698, 192.141)
  line L1328 (-52.1698, 192.141) -> (-52.1698, 197.141)
  line L1329 (-52.1698, 197.141) -> (-56.4999, 199.641)
  line L1330 (-45.8396, 199.641) -> (-50.1698, 197.141)
  line L1331 (-50.1698, 197.141) -> (-50.1698, 192.141)
  line L1332 (-50.1698, 192.141) -> (-45.8396, 189.641)
  line L1333 (-45.8396, 189.641) -> (-41.5095, 192.141)
  line L1334 (-41.5095, 192.141) -> (-41.5095, 197.141)
  line L1335 (-41.5095, 197.141) -> (-45.8396, 199.641)
  line L1336 (-35.1794, 199.641) -> (-39.5095, 197.141)
  line L1337 (-39.5095, 197.141) -> (-39.5095, 192.141)
  line L1338 (-39.5095, 192.141) -> (-35.1794, 189.641)
  line L1339 (-35.1794, 189.641) -> (-30.8493, 192.141)
  line L1340 (-30.8493, 192.141) -> (-30.8493, 197.141)
  line L1341 (-30.8493, 197.141) -> (-35.1794, 199.641)
  line L1342 (-24.5191, 199.641) -> (-28.8493, 197.141)
  line L1343 (-28.8493, 197.141) -> (-28.8493, 192.141)
  line L1344 (-28.8493, 192.141) -> (-24.5191, 189.641)
  line L1345 (-24.5191, 189.641) -> (-20.189, 192.141)
  line L1346 (-20.189, 192.141) -> (-20.189, 197.141)
  line L1347 (-20.189, 197.141) -> (-24.5191, 199.641)
  line L1348 (-13.8589, 199.641) -> (-18.189, 197.141)
  line L1349 (-18.189, 197.141) -> (-18.189, 192.141)
  line L1350 (-18.189, 192.141) -> (-13.8589, 189.641)
  line L1351 (-13.8589, 189.641) -> (-9.5287, 192.141)
  line L1352 (-9.5287, 192.141) -> (-9.5287, 197.141)
  line L1353 (-9.5287, 197.141) -> (-13.8589, 199.641)
  line L1354 (-3.1986, 199.641) -> (-7.5287, 197.141)
  line L1355 (-7.5287, 197.141) -> (-7.5287, 192.141)
  line L1356 (-7.5287, 192.141) -> (-3.1986, 189.641)
  line L1357 (-3.1986, 189.641) -> (1.1315, 192.141)
  line L1358 (1.1315, 192.141) -> (1.1315, 197.141)
  line L1359 (1.1315, 197.141) -> (-3.1986, 199.641)
  line L1360 (7.4616, 199.641) -> (3.1315, 197.141)
  line L1361 (3.1315, 197.141) -> (3.1315, 192.141)
  line L1362 (3.1315, 192.141) -> (7.4616, 189.641)
  line L1363 (7.4616, 189.641) -> (11.7918, 192.141)
  line L1364 (11.7918, 192.141) -> (11.7918, 197.141)
  line L1365 (11.7918, 197.141) -> (7.4616, 199.641)
  line L1366 (18.1219, 199.641) -> (13.7918, 197.141)
  line L1367 (13.7918, 197.141) -> (13.7918, 192.141)
  line L1368 (13.7918, 192.141) -> (18.1219, 189.641)
  line L1369 (18.1219, 189.641) -> (22.452, 192.141)
  line L1370 (22.452, 192.141) -> (22.452, 197.141)
  line L1371 (22.452, 197.141) -> (18.1219, 199.641)
  line L1372 (28.7821, 199.641) -> (24.452, 197.141)
  line L1373 (24.452, 197.141) -> (24.452, 192.141)
  line L1374 (24.452, 192.141) -> (28.7821, 189.641)
  line L1375 (28.7821, 189.641) -> (33.1123, 192.141)
  line L1376 (33.1123, 192.141) -> (33.1123, 197.141)
  line L1377 (33.1123, 197.141) -> (28.7821, 199.641)
  line L1378 (39.4424, 199.641) -> (35.1123, 197.141)
  line L1379 (35.1123, 197.141) -> (35.1123, 192.141)
  line L1380 (35.1123, 192.141) -> (39.4424, 189.641)
  line L1381 (39.4424, 189.641) -> (43.7725, 192.141)
  line L1382 (43.7725, 192.141) -> (43.7725, 197.141)
  line L1383 (43.7725, 197.141) -> (39.4424, 199.641)
  line L1384 (50.1027, 199.641) -> (45.7725, 197.141)
  line L1385 (45.7725, 197.141) -> (45.7725, 192.141)
  line L1386 (45.7725, 192.141) -> (50.1027, 189.641)
  line L1387 (50.1027, 189.641) -> (54.4328, 192.141)
  line L1388 (54.4328, 192.141) -> (54.4328, 197.141)
  line L1389 (54.4328, 197.141) -> (50.1027, 199.641)
  line L1390 (-51.1698, 208.8731) -> (-55.4999, 206.3731)
  line L1391 (-55.4999, 206.3731) -> (-55.4999, 201.3731)
  line L1392 (-55.4999, 201.3731) -> (-51.1698, 198.8731)
  line L1393 (-51.1698, 198.8731) -> (-46.8396, 201.3731)
  line L1394 (-46.8396, 201.3731) -> (-46.8396, 206.3731)
  line L1395 (-46.8396, 206.3731) -> (-51.1698, 208.8731)
  line L1396 (-40.5095, 208.8731) -> (-44.8396, 206.3731)
  line L1397 (-44.8396, 206.3731) -> (-44.8396, 201.3731)
  line L1398 (-44.8396, 201.3731) -> (-40.5095, 198.8731)
  line L1399 (-40.5095, 198.8731) -> (-36.1794, 201.3731)
  line L1400 (-36.1794, 201.3731) -> (-36.1794, 206.3731)
  line L1401 (-36.1794, 206.3731) -> (-40.5095, 208.8731)
  line L1402 (-29.8493, 208.8731) -> (-34.1794, 206.3731)
  line L1403 (-34.1794, 206.3731) -> (-34.1794, 201.3731)
  line L1404 (-34.1794, 201.3731) -> (-29.8493, 198.8731)
  line L1405 (-29.8493, 198.8731) -> (-25.5191, 201.3731)
  line L1406 (-25.5191, 201.3731) -> (-25.5191, 206.3731)
  line L1407 (-25.5191, 206.3731) -> (-29.8493, 208.8731)
  line L1408 (-19.189, 208.8731) -> (-23.5191, 206.3731)
  line L1409 (-23.5191, 206.3731) -> (-23.5191, 201.3731)
  line L1410 (-23.5191, 201.3731) -> (-19.189, 198.8731)
  line L1411 (-19.189, 198.8731) -> (-14.8589, 201.3731)
  line L1412 (-14.8589, 201.3731) -> (-14.8589, 206.3731)
  line L1413 (-14.8589, 206.3731) -> (-19.189, 208.8731)
  line L1414 (-8.5287, 208.8731) -> (-12.8589, 206.3731)
  line L1415 (-12.8589, 206.3731) -> (-12.8589, 201.3731)
  line L1416 (-12.8589, 201.3731) -> (-8.5287, 198.8731)
  line L1417 (-8.5287, 198.8731) -> (-4.1986, 201.3731)
  line L1418 (-4.1986, 201.3731) -> (-4.1986, 206.3731)
  line L1419 (-4.1986, 206.3731) -> (-8.5287, 208.8731)
  line L1420 (2.1315, 208.8731) -> (-2.1986, 206.3731)
  line L1421 (-2.1986, 206.3731) -> (-2.1986, 201.3731)
  line L1422 (-2.1986, 201.3731) -> (2.1315, 198.8731)
  line L1423 (2.1315, 198.8731) -> (6.4616, 201.3731)
  line L1424 (6.4616, 201.3731) -> (6.4616, 206.3731)
  line L1425 (6.4616, 206.3731) -> (2.1315, 208.8731)
  line L1426 (12.7918, 208.8731) -> (8.4616, 206.3731)
  line L1427 (8.4616, 206.3731) -> (8.4616, 201.3731)
  line L1428 (8.4616, 201.3731) -> (12.7918, 198.8731)
  line L1429 (12.7918, 198.8731) -> (17.1219, 201.3731)
  line L1430 (17.1219, 201.3731) -> (17.1219, 206.3731)
  line L1431 (17.1219, 206.3731) -> (12.7918, 208.8731)
  line L1432 (23.452, 208.8731) -> (19.1219, 206.3731)
  line L1433 (19.1219, 206.3731) -> (19.1219, 201.3731)
  line L1434 (19.1219, 201.3731) -> (23.452, 198.8731)
  line L1435 (23.452, 198.8731) -> (27.7821, 201.3731)
  line L1436 (27.7821, 201.3731) -> (27.7821, 206.3731)
  line L1437 (27.7821, 206.3731) -> (23.452, 208.8731)
  line L1438 (34.1123, 208.8731) -> (29.7821, 206.3731)
  line L1439 (29.7821, 206.3731) -> (29.7821, 201.3731)
  line L1440 (29.7821, 201.3731) -> (34.1123, 198.8731)
  line L1441 (34.1123, 198.8731) -> (38.4424, 201.3731)
  line L1442 (38.4424, 201.3731) -> (38.4424, 206.3731)
  line L1443 (38.4424, 206.3731) -> (34.1123, 208.8731)
  line L1444 (44.7725, 208.8731) -> (40.4424, 206.3731)
  line L1445 (40.4424, 206.3731) -> (40.4424, 201.3731)
  line L1446 (40.4424, 201.3731) -> (44.7725, 198.8731)
  line L1447 (44.7725, 198.8731) -> (49.1027, 201.3731)
  line L1448 (49.1027, 201.3731) -> (49.1027, 206.3731)
  line L1449 (49.1027, 206.3731) -> (44.7725, 208.8731)
  line L1450 (55.4328, 208.8731) -> (51.1027, 206.3731)
  line L1451 (51.1027, 206.3731) -> (51.1027, 201.3731)
  line L1452 (51.1027, 201.3731) -> (55.4328, 198.8731)
  line L1453 (55.4328, 198.8731) -> (59.7629, 201.3731)
  line L1454 (59.7629, 201.3731) -> (59.7629, 206.3731)
  line L1455 (59.7629, 206.3731) -> (55.4328, 208.8731)
  line L1456 (-56.4999, 218.1051) -> (-60.83, 215.6051)
  line L1457 (-60.83, 215.6051) -> (-60.83, 210.6051)
  line L1458 (-60.83, 210.6051) -> (-56.4999, 208.1051)
  line L1459 (-56.4999, 208.1051) -> (-52.1698, 210.6051)
  line L1460 (-52.1698, 210.6051) -> (-52.1698, 215.6051)
  line L1461 (-52.1698, 215.6051) -> (-56.4999, 218.1051)
  line L1462 (-45.8396, 218.1051) -> (-50.1698, 215.6051)
  line L1463 (-50.1698, 215.6051) -> (-50.1698, 210.6051)
  line L1464 (-50.1698, 210.6051) -> (-45.8396, 208.1051)
  line L1465 (-45.8396, 208.1051) -> (-41.5095, 210.6051)
  line L1466 (-41.5095, 210.6051) -> (-41.5095, 215.6051)
  line L1467 (-41.5095, 215.6051) -> (-45.8396, 218.1051)
  line L1468 (-35.1794, 218.1051) -> (-39.5095, 215.6051)
  line L1469 (-39.5095, 215.6051) -> (-39.5095, 210.6051)
  line L1470 (-39.5095, 210.6051) -> (-35.1794, 208.1051)
  line L1471 (-35.1794, 208.1051) -> (-30.8493, 210.6051)
  line L1472 (-30.8493, 210.6051) -> (-30.8493, 215.6051)
  line L1473 (-30.8493, 215.6051) -> (-35.1794, 218.1051)
  line L1474 (-24.5191, 218.1051) -> (-28.8493, 215.6051)
  line L1475 (-28.8493, 215.6051) -> (-28.8493, 210.6051)
  line L1476 (-28.8493, 210.6051) -> (-24.5191, 208.1051)
  line L1477 (-24.5191, 208.1051) -> (-20.189, 210.6051)
  line L1478 (-20.189, 210.6051) -> (-20.189, 215.6051)
  line L1479 (-20.189, 215.6051) -> (-24.5191, 218.1051)
  line L1480 (-13.8589, 218.1051) -> (-18.189, 215.6051)
  line L1481 (-18.189, 215.6051) -> (-18.189, 210.6051)
  line L1482 (-18.189, 210.6051) -> (-13.8589, 208.1051)
  line L1483 (-13.8589, 208.1051) -> (-9.5287, 210.6051)
  line L1484 (-9.5287, 210.6051) -> (-9.5287, 215.6051)
  line L1485 (-9.5287, 215.6051) -> (-13.8589, 218.1051)
  line L1486 (-3.1986, 218.1051) -> (-7.5287, 215.6051)
  line L1487 (-7.5287, 215.6051) -> (-7.5287, 210.6051)
  line L1488 (-7.5287, 210.6051) -> (-3.1986, 208.1051)
  line L1489 (-3.1986, 208.1051) -> (1.1315, 210.6051)
  line L1490 (1.1315, 210.6051) -> (1.1315, 215.6051)
  line L1491 (1.1315, 215.6051) -> (-3.1986, 218.1051)
  line L1492 (7.4616, 218.1051) -> (3.1315, 215.6051)
  line L1493 (3.1315, 215.6051) -> (3.1315, 210.6051)
  line L1494 (3.1315, 210.6051) -> (7.4616, 208.1051)
  line L1495 (7.4616, 208.1051) -> (11.7918, 210.6051)
  line L1496 (11.7918, 210.6051) -> (11.7918, 215.6051)
  line L1497 (11.7918, 215.6051) -> (7.4616, 218.1051)
  line L1498 (18.1219, 218.1051) -> (13.7918, 215.6051)
  line L1499 (13.7918, 215.6051) -> (13.7918, 210.6051)
  line L1500 (13.7918, 210.6051) -> (18.1219, 208.1051)
  line L1501 (18.1219, 208.1051) -> (22.452, 210.6051)
  line L1502 (22.452, 210.6051) -> (22.452, 215.6051)
  line L1503 (22.452, 215.6051) -> (18.1219, 218.1051)
  line L1504 (28.7821, 218.1051) -> (24.452, 215.6051)
  line L1505 (24.452, 215.6051) -> (24.452, 210.6051)
  line L1506 (24.452, 210.6051) -> (28.7821, 208.1051)
  line L1507 (28.7821, 208.1051) -> (33.1123, 210.6051)
  line L1508 (33.1123, 210.6051) -> (33.1123, 215.6051)
  line L1509 (33.1123, 215.6051) -> (28.7821, 218.1051)
  line L1510 (39.4424, 218.1051) -> (35.1123, 215.6051)
  line L1511 (35.1123, 215.6051) -> (35.1123, 210.6051)
  line L1512 (35.1123, 210.6051) -> (39.4424, 208.1051)
  line L1513 (39.4424, 208.1051) -> (43.7725, 210.6051)
  line L1514 (43.7725, 210.6051) -> (43.7725, 215.6051)
  line L1515 (43.7725, 215.6051) -> (39.4424, 218.1051)
  line L1516 (50.1027, 218.1051) -> (45.7725, 215.6051)
  line L1517 (45.7725, 215.6051) -> (45.7725, 210.6051)
  line L1518 (45.7725, 210.6051) -> (50.1027, 208.1051)
  line L1519 (50.1027, 208.1051) -> (54.4328, 210.6051)
  line L1520 (54.4328, 210.6051) -> (54.4328, 215.6051)
  line L1521 (54.4328, 215.6051) -> (50.1027, 218.1051)
  line L1522 (-51.1698, 227.3372) -> (-55.4999, 224.8372)
  line L1523 (-55.4999, 224.8372) -> (-55.4999, 219.8372)
  line L1524 (-55.4999, 219.8372) -> (-51.1698, 217.3372)
  line L1525 (-51.1698, 217.3372) -> (-46.8396, 219.8372)
  line L1526 (-46.8396, 219.8372) -> (-46.8396, 224.8372)
  line L1527 (-46.8396, 224.8372) -> (-51.1698, 227.3372)
  line L1528 (-40.5095, 227.3372) -> (-44.8396, 224.8372)
  line L1529 (-44.8396, 224.8372) -> (-44.8396, 219.8372)
  line L1530 (-44.8396, 219.8372) -> (-40.5095, 217.3372)
  line L1531 (-40.5095, 217.3372) -> (-36.1794, 219.8372)
  line L1532 (-36.1794, 219.8372) -> (-36.1794, 224.8372)
  line L1533 (-36.1794, 224.8372) -> (-40.5095, 227.3372)
  line L1534 (-29.8493, 227.3372) -> (-34.1794, 224.8372)
  line L1535 (-34.1794, 224.8372) -> (-34.1794, 219.8372)
  line L1536 (-34.1794, 219.8372) -> (-29.8493, 217.3372)
  line L1537 (-29.8493, 217.3372) -> (-25.5191, 219.8372)
  line L1538 (-25.5191, 219.8372) -> (-25.5191, 224.8372)
  line L1539 (-25.5191, 224.8372) -> (-29.8493, 227.3372)
  line L1540 (-19.189, 227.3372) -> (-23.5191, 224.8372)
  line L1541 (-23.5191, 224.8372) -> (-23.5191, 219.8372)
  line L1542 (-23.5191, 219.8372) -> (-19.189, 217.3372)
  line L1543 (-19.189, 217.3372) -> (-14.8589, 219.8372)
  line L1544 (-14.8589, 219.8372) -> (-14.8589, 224.8372)
  line L1545 (-14.8589, 224.8372) -> (-19.189, 227.3372)
  line L1546 (-8.5287, 227.3372) -> (-12.8589, 224.8372)
  line L1547 (-12.8589, 224.8372) -> (-12.8589, 219.8372)
  line L1548 (-12.8589, 219.8372) -> (-8.5287, 217.3372)
  line L1549 (-8.5287, 217.3372) -> (-4.1986, 219.8372)
  line L1550 (-4.1986, 219.8372) -> (-4.1986, 224.8372)
  line L1551 (-4.1986, 224.8372) -> (-8.5287, 227.3372)
  line L1552 (2.1315, 227.3372) -> (-2.1986, 224.8372)
  line L1553 (-2.1986, 224.8372) -> (-2.1986, 219.8372)
  line L1554 (-2.1986, 219.8372) -> (2.1315, 217.3372)
  line L1555 (2.1315, 217.3372) -> (6.4616, 219.8372)
  line L1556 (6.4616, 219.8372) -> (6.4616, 224.8372)
  line L1557 (6.4616, 224.8372) -> (2.1315, 227.3372)
  line L1558 (12.7918, 227.3372) -> (8.4616, 224.8372)
  line L1559 (8.4616, 224.8372) -> (8.4616, 219.8372)
  line L1560 (8.4616, 219.8372) -> (12.7918, 217.3372)
  line L1561 (12.7918, 217.3372) -> (17.1219, 219.8372)
  line L1562 (17.1219, 219.8372) -> (17.1219, 224.8372)
  line L1563 (17.1219, 224.8372) -> (12.7918, 227.3372)
  line L1564 (23.452, 227.3372) -> (19.1219, 224.8372)
  line L1565 (19.1219, 224.8372) -> (19.1219, 219.8372)
  line L1566 (19.1219, 219.8372) -> (23.452, 217.3372)
  line L1567 (23.452, 217.3372) -> (27.7821, 219.8372)
  line L1568 (27.7821, 219.8372) -> (27.7821, 224.8372)
  line L1569 (27.7821, 224.8372) -> (23.452, 227.3372)
  line L1570 (34.1123, 227.3372) -> (29.7821, 224.8372)
  line L1571 (29.7821, 224.8372) -> (29.7821, 219.8372)
  line L1572 (29.7821, 219.8372) -> (34.1123, 217.3372)
  line L1573 (34.1123, 217.3372) -> (38.4424, 219.8372)
  line L1574 (38.4424, 219.8372) -> (38.4424, 224.8372)
  line L1575 (38.4424, 224.8372) -> (34.1123, 227.3372)
  line L1576 (44.7725, 227.3372) -> (40.4424, 224.8372)
  line L1577 (40.4424, 224.8372) -> (40.4424, 219.8372)
  line L1578 (40.4424, 219.8372) -> (44.7725, 217.3372)
  line L1579 (44.7725, 217.3372) -> (49.1027, 219.8372)
  line L1580 (49.1027, 219.8372) -> (49.1027, 224.8372)
  line L1581 (49.1027, 224.8372) -> (44.7725, 227.3372)
  line L1582 (55.4328, 227.3372) -> (51.1027, 224.8372)
  line L1583 (51.1027, 224.8372) -> (51.1027, 219.8372)
  line L1584 (51.1027, 219.8372) -> (55.4328, 217.3372)
  line L1585 (55.4328, 217.3372) -> (59.7629, 219.8372)
  line L1586 (59.7629, 219.8372) -> (59.7629, 224.8372)
  line L1587 (59.7629, 224.8372) -> (55.4328, 227.3372)
  line L1588 (-56.4999, 236.5692) -> (-60.83, 234.0692)
  line L1589 (-60.83, 234.0692) -> (-60.83, 229.0692)
  line L1590 (-60.83, 229.0692) -> (-56.4999, 226.5692)
  line L1591 (-56.4999, 226.5692) -> (-52.1698, 229.0692)
  line L1592 (-52.1698, 229.0692) -> (-52.1698, 234.0692)
  line L1593 (-52.1698, 234.0692) -> (-56.4999, 236.5692)
  line L1594 (-45.8396, 236.5692) -> (-50.1698, 234.0692)
  line L1595 (-50.1698, 234.0692) -> (-50.1698, 229.0692)
  line L1596 (-50.1698, 229.0692) -> (-45.8396, 226.5692)
  line L1597 (-45.8396, 226.5692) -> (-41.5095, 229.0692)
  line L1598 (-41.5095, 229.0692) -> (-41.5095, 234.0692)
  line L1599 (-41.5095, 234.0692) -> (-45.8396, 236.5692)
  line L1600 (-35.1794, 236.5692) -> (-39.5095, 234.0692)
  line L1601 (-39.5095, 234.0692) -> (-39.5095, 229.0692)
  line L1602 (-39.5095, 229.0692) -> (-35.1794, 226.5692)
  line L1603 (-35.1794, 226.5692) -> (-30.8493, 229.0692)
  line L1604 (-30.8493, 229.0692) -> (-30.8493, 234.0692)
  line L1605 (-30.8493, 234.0692) -> (-35.1794, 236.5692)
  line L1606 (-24.5191, 236.5692) -> (-28.8493, 234.0692)
  line L1607 (-28.8493, 234.0692) -> (-28.8493, 229.0692)
  line L1608 (-28.8493, 229.0692) -> (-24.5191, 226.5692)
  line L1609 (-24.5191, 226.5692) -> (-20.189, 229.0692)
  line L1610 (-20.189, 229.0692) -> (-20.189, 234.0692)
  line L1611 (-20.189, 234.0692) -> (-24.5191, 236.5692)
  line L1612 (-13.8589, 236.5692) -> (-18.189, 234.0692)
  line L1613 (-18.189, 234.0692) -> (-18.189, 229.0692)
  line L1614 (-18.189, 229.0692) -> (-13.8589, 226.5692)
  line L1615 (-13.8589, 226.5692) -> (-9.5287, 229.0692)
  line L1616 (-9.5287, 229.0692) -> (-9.5287, 234.0692)
  line L1617 (-9.5287, 234.0692) -> (-13.8589, 236.5692)
  line L1618 (-3.1986, 236.5692) -> (-7.5287, 234.0692)
  line L1619 (-7.5287, 234.0692) -> (-7.5287, 229.0692)
  line L1620 (-7.5287, 229.0692) -> (-3.1986, 226.5692)
  line L1621 (-3.1986, 226.5692) -> (1.1315, 229.0692)
  line L1622 (1.1315, 229.0692) -> (1.1315, 234.0692)
  line L1623 (1.1315, 234.0692) -> (-3.1986, 236.5692)
  line L1624 (7.4616, 236.5692) -> (3.1315, 234.0692)
  line L1625 (3.1315, 234.0692) -> (3.1315, 229.0692)
  line L1626 (3.1315, 229.0692) -> (7.4616, 226.5692)
  line L1627 (7.4616, 226.5692) -> (11.7918, 229.0692)
  line L1628 (11.7918, 229.0692) -> (11.7918, 234.0692)
  line L1629 (11.7918, 234.0692) -> (7.4616, 236.5692)
  line L1630 (18.1219, 236.5692) -> (13.7918, 234.0692)
  line L1631 (13.7918, 234.0692) -> (13.7918, 229.0692)
  line L1632 (13.7918, 229.0692) -> (18.1219, 226.5692)
  line L1633 (18.1219, 226.5692) -> (22.452, 229.0692)
  line L1634 (22.452, 229.0692) -> (22.452, 234.0692)
  line L1635 (22.452, 234.0692) -> (18.1219, 236.5692)
  line L1636 (28.7821, 236.5692) -> (24.452, 234.0692)
  line L1637 (24.452, 234.0692) -> (24.452, 229.0692)
  line L1638 (24.452, 229.0692) -> (28.7821, 226.5692)
  line L1639 (28.7821, 226.5692) -> (33.1123, 229.0692)
  line L1640 (33.1123, 229.0692) -> (33.1123, 234.0692)
  line L1641 (33.1123, 234.0692) -> (28.7821, 236.5692)
  line L1642 (39.4424, 236.5692) -> (35.1123, 234.0692)
  line L1643 (35.1123, 234.0692) -> (35.1123, 229.0692)
  line L1644 (35.1123, 229.0692) -> (39.4424, 226.5692)
  line L1645 (39.4424, 226.5692) -> (43.7725, 229.0692)
  line L1646 (43.7725, 229.0692) -> (43.7725, 234.0692)
  line L1647 (43.7725, 234.0692) -> (39.4424, 236.5692)
  line L1648 (50.1027, 236.5692) -> (45.7725, 234.0692)
  line L1649 (45.7725, 234.0692) -> (45.7725, 229.0692)
  line L1650 (45.7725, 229.0692) -> (50.1027, 226.5692)
  line L1651 (50.1027, 226.5692) -> (54.4328, 229.0692)
  line L1652 (54.4328, 229.0692) -> (54.4328, 234.0692)
  line L1653 (54.4328, 234.0692) -> (50.1027, 236.5692)